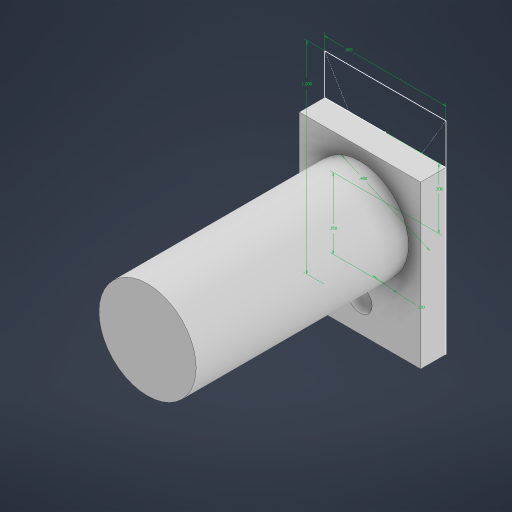
# Autodesk Inventor part: FRONT_AXEL
Saved by Autodesk Inventor 2024.1 (Build 281209000, 209)
## iProperties
Created: 2023-11-05
Part Number: FRONT_AXEL
Material: Generic
Document SubType Name: Modeling
Designer: jerem
Density: 1 g/cm^3
Appearance: Default
Author: jerem
Autodesk Inventor part; units mm, degrees
ref_plane "YZ Plane" through (0, 0, 0) normal (1, 0, 0) x (0, 1, 0)
ref_plane "XZ Plane" through (0, 0, 0) normal (0, 1, 0) x (-1, 0, 0)
ref_plane "XY Plane" through (0, 0, 0) normal (0, 0, 1) x (1, 0, 0)
sketch "Sketch1" plane through (0, 0, 0) normal (0, 0, 1) x (1, 0, 0)
  line L0 (7.62, 12.7) -> (-7.62, 12.7)
  line L1 (-7.62, 12.7) -> (-7.62, -12.7)
  line L2 (-7.62, -12.7) -> (7.62, -12.7)
  line L3 (7.62, -12.7) -> (7.62, 12.7)
  line L4 (7.62, 12.7) -> (-7.62, -12.7) construction
  line L5 (-7.62, 12.7) -> (7.62, -12.7) construction
  circle A0 centre (0, 0) radius 6.096
  circle A1 centre (0, -8.89) radius 1.524
  line L6 (7.62, 7.62) -> (-7.62, 7.62)
  point P0 (0, 7.62)
  dimension "d0" = 12.192
  dimension "d1" = 15.24
  dimension "d2" = 25.4
  dimension "d7" = 3.048
  dimension "d8" = 8.89
  dimension "d10" = 7.62
  constraints: 14 end point, 3 midpoint, 2 centre point, 2 parallel, 2 perpendicular, 2 point on line, 1 coincident, 1 horizontal
  measures "d0" diameter of A0
  measures "d1" distance of L0.start L0.end
  measures "d2" distance of L0.end L1.end
  measures "d7" diameter of A1
  measures "d8" distance of A1.centre point (0, 0)
  measures "d10" distance of A0.centre point (0, 7.62)
extrude "Extrusion1" add sketch "Sketch1" along normal blind 3.175 contours L3 L2 L1 L6 | A0
extrude "Extrusion2" add sketch "Sketch1" along normal blind 26.67 from surface at 3.175 contours A0
body "Solid1"
